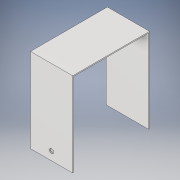
# Autodesk Inventor part: MAN_BASIS_THIRD_STRUCTURE
Saved by Autodesk Inventor 2019 (Build 230136000, 136)
## iProperties
Created: 2021-03-07
Part Number: MAN_BASIS_THIRD_STRUCTURE
Material: ABS Plastic
Document SubType Name: Modeling
Designer: DOMEK
Density: 1.06 g/cm^3
Appearance: Smooth - White
Author: DOMEK
Autodesk Inventor part; units mm, degrees
ref_plane "YZ Plane" through (0, 0, 0) normal (1, 0, 0) x (0, 1, 0)
ref_plane "XZ Plane" through (0, 0, 0) normal (0, 1, 0) x (-1, 0, 0)
ref_plane "XY Plane" through (0, 0, 0) normal (0, 0, 1) x (1, 0, 0)
sketch "Sketch3" plane through (0, 0, 0) normal (1, 0, 0) x (0, 1, 0)
  line L0 (0, 0) -> (80, 0)
  line L1 (80, 0) -> (80, 73)
  line L2 (80, 73) -> (0, 73)
  line L3 (0, 73) -> (0, 0)
  dimension "d8" = 80
  dimension "d9" = 73
  constraints: 8 end point, 2 parallel, 1 horizontal, 1 perpendicular
  measures "d8" distance of L2.end L1.end
  measures "d9" distance of L1.end L0.end
extrude "Extrusion3" add sketch "Sketch3" along normal blind 40
shell "Shell1" thickness 1 removed faces 3 at (40, 53.3333, 24.3333) at (0, 53.3333, 24.3333) at (26.6667, 0, 48.6667)
sketch "Sketch4" plane through (0, 0, 73) normal (0, 0, 1) x (1, 0, 0)
  line L0 (0, 0) -> (40, 0) projected
  line L1 (0, 80) -> (40, 80) projected
  circle A0 centre (20, 8.0945) radius 2
  dimension "d13" = 4
  constraints: 1 centre point
  measures "d13" diameter of A0
extrude "Extrusion4" cut sketch "Sketch4" against normal blind 1
body "Solid2"
